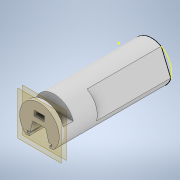
# Autodesk Inventor part: lamp
Saved by Autodesk Inventor 2020 (Build 240168000, 168)
## iProperties
Created: 2022-10-15
Part Number: lamp
Material: Типовые
Document SubType Name: Modeling
Designer: zigma
Density: 1 g/cm^3
Appearance: По умолчанию
Author: zigma
Autodesk Inventor part; units mm, degrees
ref_plane "YZ Plane" through (0, 0, 0) normal (1, 0, 0) x (0, 1, 0)
ref_plane "XZ Plane" through (0, 0, 0) normal (0, 1, 0) x (-1, 0, 0)
ref_plane "XY Plane" through (0, 0, 0) normal (0, 0, 1) x (1, 0, 0)
sketch "Эскиз1" plane through (0, 0, 0) normal (0, 0, 1) x (1, 0, 0)
  arc A0 (47.2167, -13.0271) -> (19.1654, -13.0271) centre (33.1911, 1.2306) ccw
  line L0 (26.6911, 1.9729) -> (39.6911, 1.9729)
  line L1 (39.6911, 1.9729) -> (42.6385, -9.0271)
  line L2 (33.1911, 1.9729) -> (33.1911, -13.0271) construction
  line L3 (26.6911, 1.9729) -> (23.7436, -9.0271)
  line L4 (22.6718, -13.0271) -> (22.6718, -11.0271)
  line L5 (22.6718, -11.0271) -> (20.6718, -11.0271)
  line L6 (20.6718, -11.0271) -> (20.6718, -9.0271)
  line L7 (20.6718, -9.0271) -> (23.7436, -9.0271)
  line L8 (43.7103, -13.0271) -> (43.7103, -11.0271)
  line L9 (43.7103, -11.0271) -> (45.7103, -11.0271)
  line L10 (45.7103, -11.0271) -> (45.7103, -9.0271)
  line L11 (45.7103, -9.0271) -> (42.6385, -9.0271)
  line L12 (19.1654, -13.0271) -> (22.6718, -13.0271)
  line L13 (43.7103, -13.0271) -> (47.2167, -13.0271)
  point P0 (19.1654, -13.0271)
  dimension "d3" = 13
  dimension "d4" = 105
  dimension "d5" = 15
  dimension "d6" = 40
  dimension "d44" = 2
  dimension "d45" = 2
  dimension "d46" = 2
  dimension "d47" = 3.5064
  constraints: 28 end point, 5 symmetric about line, 3 horizontal, 3 perpendicular, 2 point on circle, 2 vertical, 1 centre point, 1 midpoint, 1 other
  measures "d3" distance of L0.start L0.end
  measures "d4" angle of L0 L1
  measures "d5" distance from line of A0.end L0
  measures "d6" diameter of A0
  measures "d44" distance of L4.start L4.end
  measures "d45" distance of L4.end L5.end
  measures "d46" distance of L5.end L6.end
  measures "d47" distance of L4.start A0.end
extrude "Выдавливание1" add sketch "Эскиз1" along normal blind 200
sketch "Эскиз3" plane through (0, 0, 200) normal (0, 0, 1) x (1, 0, 0)
  arc A0 (47.2167, -13.0271) -> (19.1654, -13.0271) centre (33.1911, 1.2306) ccw projected
  circle A1 centre (33.1911, 1.2306) radius 20
  point P0 (0, 0)
  point P1 (19.1654, -13.0271)
  constraints: 1 coincident, 3 other
extrude "Выдавливание3" add sketch "Эскиз3" along normal blind 15
sketch "Эскиз5" plane through (33.1911, 1.2306, 215) normal (0, 0, 1) x (1, 0, 0)
  circle A0 centre (0, -12) radius 6
  circle A1 centre (0, 0) radius 20 construction
  circle A2 centre (0, 0) radius 18 construction
  circle A3 centre (0, 0) radius 20 construction
  line L0 (0, -20) -> (0, 0)
  point P0 (-33.1911, -1.2306)
  dimension "d38" = 12
  dimension "d39" = 2
  constraints: 3 centre point, 2 end point, 1 coincident, 1 point on line, 1 tangent, 1 vertical, 1 vertical alignment, 2 other
  measures "d38" diameter of A0
  measures "d39" radial gap between concentric circles of A1 A2
extrude "Выдавливание5" cut sketch "Эскиз5" against normal blind 15
sketch "Эскиз6" plane through (0, 0, 0) normal (0, 0, -1) x (-1, 0, 0)
  arc A0 (-19.1654, -13.0271) -> (-47.2167, -13.0271) centre (-33.1911, 1.2306) ccw
  arc A1 (-19.1654, -13.0271) -> (-47.2167, -13.0271) centre (-33.1911, 1.2306) ccw projected
  line L0 (-19.1654, -13.0271) -> (-22.6718, -13.0271) projected
  line L1 (-19.1654, -13.0271) -> (-22.6718, -13.0271)
  line L2 (-22.6718, -13.0271) -> (-22.6718, -11.0271) projected
  line L3 (-22.6718, -13.0271) -> (-22.6718, -11.0271)
  line L4 (-22.6718, -11.0271) -> (-20.6718, -11.0271) projected
  line L5 (-22.6718, -11.0271) -> (-20.6718, -11.0271)
  line L6 (-20.6718, -11.0271) -> (-20.6718, -9.0271) projected
  line L7 (-20.6718, -11.0271) -> (-20.6718, -9.0271)
  line L8 (-20.6718, -9.0271) -> (-23.7436, -9.0271) projected
  line L9 (-20.6718, -9.0271) -> (-23.7436, -9.0271)
  line L10 (-23.7436, -9.0271) -> (-26.6911, 1.9729) projected
  line L11 (-23.7436, -9.0271) -> (-26.6911, 1.9729)
  line L12 (-39.6911, 1.9729) -> (-42.6385, -9.0271) projected
  line L13 (-26.6911, 1.9729) -> (-39.6911, 1.9729)
  line L14 (-39.6911, 1.9729) -> (-42.6385, -9.0271)
  line L15 (-42.6385, -9.0271) -> (-45.7103, -9.0271) projected
  line L16 (-42.6385, -9.0271) -> (-45.7103, -9.0271)
  line L17 (-45.7103, -9.0271) -> (-45.7103, -11.0271) projected
  line L18 (-45.7103, -9.0271) -> (-45.7103, -11.0271)
  line L19 (-45.7103, -11.0271) -> (-43.7103, -11.0271) projected
  line L20 (-45.7103, -11.0271) -> (-43.7103, -11.0271)
  line L21 (-43.7103, -11.0271) -> (-43.7103, -13.0271) projected
  line L22 (-43.7103, -11.0271) -> (-43.7103, -13.0271)
  line L23 (-43.7103, -13.0271) -> (-47.2167, -13.0271)
  point P0 (0, 0)
  constraints: 26 end point, 7 perpendicular, 4 collinear, 2 point on circle, 1 centre point, 1 concentric, 1 horizontal, 1 parallel
extrude "Выдавливание6" add sketch "Эскиз6" along normal blind 12
sketch "Эскиз7" plane through (0, 0, -12) normal (0, 0, -1) x (-1, 0, 0)
  arc A0 (-14.0248, 6.9449) -> (-52.3574, 6.9449) centre (-33.1911, 1.2306) ccw projected
  circle A1 centre (-33.1911, 1.2306) radius 20
  arc A2 (-19.1654, -13.0271) -> (-47.2167, -13.0271) centre (-33.1911, 1.2306) ccw projected
  circle A3 centre (-33.1911, 1.2306) radius 20 projected
  line L0 (-52.4096, -4.3055) -> (-42.7971, 18.7726)
  point P0 (0, 0)
  point P1 (-42.7971, 18.7726)
  point P2 (-52.3574, 6.9449)
  dimension "d50" = 25
  constraints: 2 end point, 2 point on circle, 1 centre point, 1 coincident, 1 concentric
  measures "d50" distance of L0.start L0.end
extrude "Выдавливание7" cut sketch "Эскиз7" against normal blind 75 contours L0 A1 A0 picked at (-49.4328, 5.896)
sketch "Эскиз8" plane through (0, 0, -12) normal (0, 0, -1) x (-1, 0, 0)
  arc A0 (-14.0248, 6.9449) -> (-52.3574, 6.9449) centre (-33.1911, 1.2306) ccw projected
  arc A1 (-52.4096, -4.3055) -> (-42.7971, 18.7726) centre (-33.1911, 1.2306) ccw
  line L0 (-42.7971, 18.7726) -> (-52.4096, -4.3055)
  line L1 (-39.8961, 17.9351) -> (-49.5086, -5.143)
  arc A2 (-15.4012, 3.9729) -> (-39.8961, 17.9351) centre (-33.1911, 1.2306) ccw
  line L2 (-39.6911, 1.9729) -> (-26.6747, 1.9729)
  line L3 (-43.0035, 3.9729) -> (-15.4012, 3.9729)
  line L4 (-43.0035, 3.9729) -> (-47.2008, -6.1043)
  line L5 (-49.5086, -5.143) -> (-47.2008, -6.1043)
  point P0 (0, 0)
  point P1 (-40.9509, 18.0036)
  dimension "d53" = 3
  dimension "d54" = 25
  dimension "d55" = 2
  dimension "d56" = 2.5
  dimension "d57" = 2
  constraints: 12 end point, 4 point on circle, 3 parallel, 2 centre point, 1 coincident, 1 concentric, 1 horizontal
  measures "d53" distance between parallel lines of L0 L1
  measures "d54" distance of L1.start L1.end
  measures "d55" distance between parallel lines of L2 L3
  measures "d56" distance between parallel lines of L1 L4
  measures "d57" radial gap between concentric circles of A1 A2
extrude "Выдавливание8" cut sketch "Эскиз8" against normal blind 75 contours A2 L3 L4 L5 L1
ref_plane "РабПлоскость3" through (33.1911, 1.2306, 101.5) normal (0, 0, 1) x (1, 0, 0)
sketch "Эскиз11" plane through (33.1911, 1.2306, 215) normal (0, 0, 1) x (1, 0, 0)
  circle A0 centre (0, 0) radius 20 projected
  circle A1 centre (0, 0) radius 20
  point P0 (-33.1911, -1.2306)
  constraints: 1 centre point, 1 coincident, 1 concentric
extrude "Выдавливание11" cut sketch "Эскиз11" against normal up to surface (113.5 mm away)
ref_plane "РабПлоскость4" through (33.1911, 1.2306, 96.5) normal (0, 0, 1) x (1, 0, 0)
sketch "Эскиз12" plane through (33.1911, 1.2306, 96.5) normal (0, 0, 1) x (1, 0, 0)
  arc A0 (9.6061, 17.5421) -> (-14.0257, -14.2577) centre (0, 0) ccw projected
  circle A1 centre (0, 0) radius 20
  line L0 (-36.0884, 6) -> (47.8773, 6)
  point P0 (-33.1911, -1.2306)
  point P1 (-19.0788, 6)
  point P2 (19.0788, 6)
  point P3 (9.6061, 17.5421)
  dimension "d75" = 6
  constraints: 2 end point, 1 centre point, 1 coincident, 1 concentric, 1 horizontal
  measures "d75" distance from line of A1.centre L0
extrude "Выдавливание12" cut sketch "Эскиз12" against normal blind 10 contours A1 L0 A0 picked at (3.202, 9.8473)
sketch "Эскиз13" plane through (33.1911, 1.2306, 101.5) normal (0, 0, 1) x (1, 0, 0)
  circle A0 centre (0, 0) radius 20
  arc A1 (14.0257, -14.2577) -> (-14.0257, -14.2577) centre (0, 0) ccw projected
  line L0 (0, 0) -> (0, 20)
  arc A2 (9.6061, 17.5421) -> (-14.0257, -14.2577) centre (0, 0) ccw projected
  line L1 (-5, 11) -> (5, 11)
  line L2 (5, 11) -> (5, 6)
  line L3 (5, 6) -> (-5, 6)
  line L4 (-5, 6) -> (-5, 11)
  point P0 (-33.1911, -1.2306)
  point P1 (0, 11)
  dimension "d78" = 10
  dimension "d79" = 5
  dimension "d80" = 6
  constraints: 10 end point, 2 parallel, 2 point on circle, 1 coincident, 1 horizontal, 1 midpoint, 1 perpendicular, 1 point on line, 3 other
  measures "d78" distance of L2.end L3.end
  measures "d79" distance of L1.end L2.end
  measures "d80" distance from line of point (0, 0) L3
extrude "Выдавливание13" cut sketch "Эскиз13" against normal blind 5 contours L3 L4 L1 L0 | L0 L1 L2 L3
sketch "Эскиз14" plane through (26.6911, 1.9729, -12) normal (0, -1, 0) x (1, 0, 0)
  line L0 (11.5, 8) -> (1.5, 8)
  line L1 (1.5, 8) -> (1.5, 3)
  line L2 (1.5, 3) -> (11.5, 3)
  line L3 (11.5, 3) -> (11.5, 8)
  line L4 (13, 0) -> (0, 0) construction
  line L5 (13, 0) -> (0, 0) construction
  line L6 (6.5, 27.1323) -> (6.5, 0) construction
  point P0 (-26.6911, 12)
  point P1 (6.5, 3)
  dimension "d83" = 10
  dimension "d84" = 5
  dimension "d85" = 3
  constraints: 12 end point, 3 equal length, 2 midpoint, 1 horizontal, 1 perpendicular, 1 point on line, 1 vertical
  measures "d83" distance of L2.end L1.end
  measures "d84" distance of L1.end L0.end
  measures "d85" distance between parallel lines of L4 L2
extrude "Выдавливание14" cut sketch "Эскиз14" against normal blind 4
sketch "Эскиз15" plane through (0, 0, -12) normal (0, 0, -1) x (-1, 0, 0)
  arc A0 (-19.1654, -13.0271) -> (-42.7971, 18.7726) centre (-33.1911, 1.2306) ccw projected
  arc A1 (-42.7971, 18.7726) -> (-52.4096, -4.3055) centre (-33.1911, 1.2306) ccw projected
  line L0 (-47.2008, -6.1043) -> (-49.5086, -5.143) projected
  line L1 (-49.5086, -5.143) -> (-47.2008, -6.1043)
  line L2 (-15.4012, 3.9729) -> (-43.0035, 3.9729) projected
  line L3 (-47.2008, -6.1043) -> (-43.0035, 3.9729)
  line L4 (-43.0035, 3.9729) -> (-15.4012, 3.9729)
  line L5 (-49.5086, -5.143) -> (-39.8961, 17.9351) projected
  line L6 (-49.5086, -5.143) -> (-39.8961, 17.9351)
  line L7 (-47.2167, -13.0271) -> (-43.7103, -13.0271) projected
  line L8 (-47.2167, -13.0271) -> (-43.7103, -13.0271)
  line L9 (-43.7103, -13.0271) -> (-43.7103, -11.0271) projected
  line L10 (-43.7103, -13.0271) -> (-43.7103, -11.0271)
  line L11 (-43.7103, -11.0271) -> (-45.7103, -11.0271) projected
  line L12 (-43.7103, -11.0271) -> (-45.7103, -11.0271)
  line L13 (-45.7103, -11.0271) -> (-45.7103, -9.0271) projected
  line L14 (-45.7103, -11.0271) -> (-45.7103, -9.0271)
  line L15 (-45.7103, -9.0271) -> (-42.6385, -9.0271) projected
  line L16 (-45.7103, -9.0271) -> (-42.6385, -9.0271)
  line L17 (-42.6385, -9.0271) -> (-39.6911, 1.9729) projected
  line L18 (-42.6385, -9.0271) -> (-39.6911, 1.9729)
  line L19 (-39.6911, 1.9729) -> (-26.6911, 1.9729) projected
  line L20 (-39.6911, 1.9729) -> (-26.6911, 1.9729)
  line L21 (-23.7436, -9.0271) -> (-20.6718, -9.0271) projected
  line L22 (-26.6911, 1.9729) -> (-23.7436, -9.0271)
  line L23 (-23.7436, -9.0271) -> (-20.6718, -9.0271)
  line L24 (-20.6718, -9.0271) -> (-20.6718, -11.0271) projected
  line L25 (-20.6718, -9.0271) -> (-20.6718, -11.0271)
  line L26 (-22.6718, -11.0271) -> (-22.6718, -13.0271) projected
  line L27 (-20.6718, -11.0271) -> (-22.6718, -11.0271)
  line L28 (-22.6718, -11.0271) -> (-22.6718, -13.0271)
  line L29 (-22.6718, -13.0271) -> (-19.1654, -13.0271)
  arc A2 (-15.4012, 3.9729) -> (-39.8961, 17.9351) centre (-33.1911, 1.2306) ccw
  arc A3 (-15.4012, 3.9729) -> (-39.8961, 17.9351) centre (-33.1911, 1.2306) ccw projected
  line L30 (-52.4096, -4.3055) -> (-42.7971, 18.7726)
  arc A4 (-52.4096, -4.3055) -> (-47.2167, -13.0271) centre (-33.1911, 1.2306) ccw
  arc A5 (-19.1654, -13.0271) -> (-42.7971, 18.7726) centre (-33.1911, 1.2306) ccw
  point P0 (0, 0)
  constraints: 36 end point, 8 perpendicular, 7 collinear, 6 point on circle, 3 centre point, 2 coincident, 2 point on line, 1 concentric, 1 horizontal
